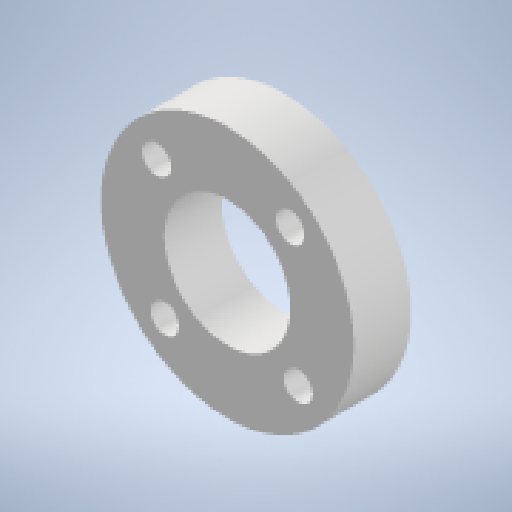
# Autodesk Inventor part: gear ring
Saved by Autodesk Inventor 2023 (Build 270158000, 158)
## iProperties
Created: 2023-11-14
Part Number: gear ring
Material: Generic
Document SubType Name: Modeling
Designer: Nate
Density: 1 g/cm^3
Appearance: Default
Author: Nate
Autodesk Inventor part; units mm, degrees
ref_plane "YZ Plane" through (0, 0, 0) normal (1, 0, 0) x (0, 1, 0)
ref_plane "XZ Plane" through (0, 0, 0) normal (0, 1, 0) x (-1, 0, 0)
ref_plane "XY Plane" through (0, 0, 0) normal (0, 0, 1) x (1, 0, 0)
sketch "Sketch1" plane through (0, 0, 0) normal (0, 0, 1) x (1, 0, 0)
  circle A0 centre (0, 0) radius 3.5
  circle A1 centre (0, 0) radius 7
  circle A2 centre (3.9313, -3.4792) radius 0.7937
  circle A3 centre (3.4792, 3.9313) radius 0.7937
  circle A4 centre (-3.9313, 3.4792) radius 0.7937
  circle A5 centre (-3.4792, -3.9313) radius 0.7937
  dimension "d0" = 7
  dimension "d1" = 14
  dimension "d2" = 1.5875
  dimension "d3" = 0.956
  dimension "d6" = 360
  dimension "d10" = 0.956
  dimension "d11" = 0.956
  dimension "d12" = 0.956
  dimension "d13" = 5.8368
  dimension "d14" = 5.8368
  dimension "d15" = 5.8368
  constraints: 6 centre point, 4 coincident, 11 other
  measures "d0" diameter of A0
  measures "d1" diameter of A1
  measures "d2" diameter of A2
extrude "Extrusion1" add sketch "Sketch1" along normal blind 3.175
body "Solid1"
